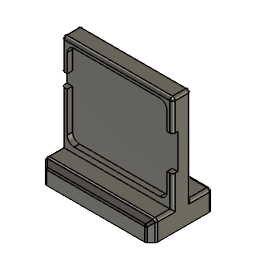
gnss-mount (Autodesk Fusion 360 design; units mm, degrees)
part number: 2026-07-21-16-58-32-799
Autodesk Fusion 360 part; units mm, degrees
sketch "Sketch1" plane through (0, 0, 0) normal (0, 0, 1) x (1, 0, 0)
  line L0 (40, 22.7) -> (40, 1.5)
  line L1 (41.5, 24.2) -> (41.5, 0)
  line L2 (1.5, 1.5) -> (1.5, 22.7)
  line L3 (41.5, 0) -> (0, 0)
  line L4 (1.5, 22.7) -> (40, 22.7)
  line L5 (0, 24.2) -> (41.5, 24.2)
  line L6 (40, 1.5) -> (1.5, 1.5)
  line L7 (-47.8655, -10.4699) -> (-48.8655, -12.202)
  line L8 (0, 0) -> (0, 24.2)
  line L9 (-48.8655, 12.202) -> (-47.8655, 10.4699)
  point P0 (-0.0762, -5.2837)
  dimension "d87" = -1.5
  dimension "d2" = 38.5
  dimension "d3" = 21.2
  dimension "d4" = 1.7321
  dimension "d5" = 120
  dimension "d6" = 47.8655
  dimension "d7" = 10.4699
  dimension "d8" = 10.4699
  dimension "d9" = 0.0762
  dimension "d10" = 5.2837
  constraint perpendicular L2 L4
  constraint perpendicular L0 L6
  constraint perpendicular L0 L4
  constraint coincident L3.end L8.start
  constraint vertical L8
  constraint vertical L7.end L9.start
  constraint vertical L7.start L9.end
  constraint equal L7 L9
  measures "d2" distance of L2.end L0.start
  measures "d3" distance of L2.end L2.start
  measures "d4" vertical distance of L9.start L9.end
  measures "d5" angle of L7 L9
  measures "d6" distance of L9.end L8
  measures "d7" distance of L7.start L3
  measures "d8" distance of L9.end L3
  measures "d9" distance of P0 L8
  measures "d10" distance of P0 L3
extrude "Extrude1" add sketch "Sketch1" against normal blind 5
sketch "Sketch2" plane through (0, 0, 0) normal (0, 0, 1) x (1, 0, 0)
  line L0 (0, 0) -> (41.5, 0)
  line L1 (41.5, 0) -> (41.5, 24.2)
  line L2 (41.5, 24.2) -> (0, 24.2)
  line L3 (0, 24.2) -> (0, 0)
  dimension "d16" = 41.5
  dimension "d17" = 24.2
  constraint horizontal L0
  constraint vertical L1
  constraint horizontal L2
  constraint vertical L3
  constraint coincident L0.start L3.end
  measures "d16" distance of L0.start L0.end
  measures "d17" distance of L0.start L2.end
extrude "Extrude2" add sketch "Sketch2" along normal blind 2.5
sketch "Sketch3" plane through (0, 0, 2.5) normal (0, 0, 1) x (-1, 0, 0)
  line L0 (0, -24.2) -> (0, 0)
  line L1 (0, 0) -> (-41.5, 0)
  line L2 (-41.5, 0) -> (-41.5, -24.2)
  line L3 (-41.5, -24.2) -> (0, -24.2)
  line L4 (0, -15) -> (-41.5, -15)
  line L5 (-41.5, -15) -> (-41.5, -10)
  line L6 (-41.5, -10) -> (0, -10)
  line L7 (0, -10) -> (0, -15)
  dimension "d20" = 41.5
  dimension "d21" = 5
  dimension "d22" = 9.2
  constraint horizontal L4
  constraint vertical L5
  constraint horizontal L6
  constraint vertical L7
  constraint coincident L0 L4.start
  measures "d20" distance of L4.start L4.end
  measures "d21" distance of L4.start L6.end
  measures "d22" distance of L3 L4
extrude "Extrude3" add sketch "Sketch3" along normal blind 36 contours L0 L2 L4 L5 L6 L7
sketch "Sketch4" plane through (0, 10, 0) normal (0, -1, 0) x (1, 0, 0)
  line L0 (0, 2.5) -> (41.5, 2.5)
  line L1 (41.5, 2.5) -> (41.5, 38.5)
  line L2 (41.5, 38.5) -> (0, 38.5)
  line L3 (0, 38.5) -> (0, 2.5)
  line L4 (4.7, 36.5) -> (36.8, 36.5)
  line L5 (39.4, 33.9) -> (39.4, 7.2)
  line L6 (36.8, 4.6) -> (4.7, 4.6)
  line L7 (2.1, 7.2) -> (2.1, 33.9)
  arc A0 (4.7, 36.5) -> (2.1, 33.9) centre (4.7, 33.9) ccw
  arc A1 (39.4, 33.9) -> (36.8, 36.5) centre (36.8, 33.9) ccw
  arc A2 (2.1, 7.2) -> (4.7, 4.6) centre (4.7, 7.2) ccw
  arc A3 (36.8, 4.6) -> (39.4, 7.2) centre (36.8, 7.2) ccw
  line L8 (31.4, 27.05) -> (47.4, 27.05)
  line L9 (47.4, 27.05) -> (47.4, 14.05)
  line L10 (47.4, 14.05) -> (31.4, 14.05)
  line L11 (31.4, 14.05) -> (31.4, 27.05)
  line L12 (31.4, 27.05) -> (47.4, 14.05) construction
  line L13 (47.4, 27.05) -> (31.4, 14.05) construction
  line L14 (-2, 27) -> (5, 27)
  line L15 (5, 27) -> (5, 22)
  line L16 (5, 22) -> (-2, 22)
  line L17 (-2, 22) -> (-2, 27)
  point P0 (2.1, 36.5)
  point P1 (39.4, 36.5)
  point P2 (2.1, 4.6)
  point P3 (39.4, 20.55)
  dimension "d25" = 37.3
  dimension "d26" = 31.9
  dimension "d27" = 2.1
  dimension "d28" = 2
  dimension "d29" = 2.6
  dimension "d30" = 2.6
  dimension "d31" = 2.6
  dimension "d32" = 2.6
  dimension "d33" = 16
  dimension "d34" = 13
  dimension "d35" = 2
  dimension "d36" = 19.5
  dimension "d37" = 11.5
  dimension "d38" = 5
  constraint horizontal L4
  constraint vertical L5
  constraint horizontal L6
  constraint vertical L7
  constraint coincident P0 L4
  constraint coincident P0 L7
  constraint tangent L4 A0
  constraint tangent L7 A0
  constraint coincident P1 L4
  constraint coincident P1 L5
  constraint tangent L4 A1
  constraint tangent L5 A1
  constraint coincident P2 L6
  constraint coincident P2 L7
  constraint tangent L6 A2
  constraint tangent L7 A2
  constraint tangent L6 A3
  constraint tangent L5 A3
  constraint horizontal L8
  constraint perpendicular L8 L9
  constraint parallel L8 L10
  constraint parallel L9 L11
  constraint coincident L12 P3
  constraint coincident L13 P3
  constraint midpoint L5 P3
  constraint horizontal L14
  constraint vertical L15
  constraint horizontal L16
  constraint vertical L17
  measures "d25" distance of P0 P1
  measures "d26" distance of P0 P2
  measures "d27" distance of L3 L7
  measures "d28" distance of L2 L4
  measures "d29" radius of A0
  measures "d30" radius of A1
  measures "d31" radius of A2
  measures "d32" radius of A3
  measures "d33" distance of L9.end L10.end
  measures "d34" distance of L8.end L9.end
  measures "d35" distance of L3 L17
  measures "d36" distance of L0 L16
  measures "d37" distance of L2 L14
  measures "d38" distance of L3 L15
extrude "Extrude4" add sketch "Sketch4" along normal blind 2 contours L0 L1 L3 L5 L6 L7 A2 A3 L10 L16 | L1 L2 L3 L4 L5 L7 A0 A1 L8 L14
fillet "Fillet1" radius 1 10 edges at (20.75, 15, 38.5) (20.75, 8, 38.5) (41.5, 11.5, 38.5) (0, 11.5, 38.5) (0, 8, 32.75) (0, 8, 12.25) (0, 15, 20.5) (41.5, 8, 32.775) (41.5, 8, 8.275) (41.5, 15, 20.5)
chamfer "Chamfer1" distance 2 angle 45 6 edges at (20.75, 0, 2.5) (20.75, 24.2, 2.5) (0, 0, -1.25) (0, 24.2, -1.25) (41.5, 0, -1.25) (41.5, 24.2, -1.25)
fillet "Fillet2" radius 1 10 edges at (20.75, 2, 2.5) (0, 5.5, 2.5) (1, 1, 1.5) (0, 2, -1.25) (2, 0, -2.25) (20.75, 0, 0.5) (40.5, 1, 1.5) (39.5, 0, -2.25) (41.5, 5.5, 2.5) (41.5, 2, -1.25)
fillet "Fillet3" radius 1 10 edges at (41.5, 18.1, 2.5) (20.75, 22.2, 2.5) (41.5, 22.2, -1.25) (40.5, 23.2, 1.5) (39.5, 24.2, -2.25) (20.75, 24.2, 0.5) (0, 18.1, 2.5) (1, 23.2, 1.5) (0, 22.2, -1.25) (2, 24.2, -2.25)
